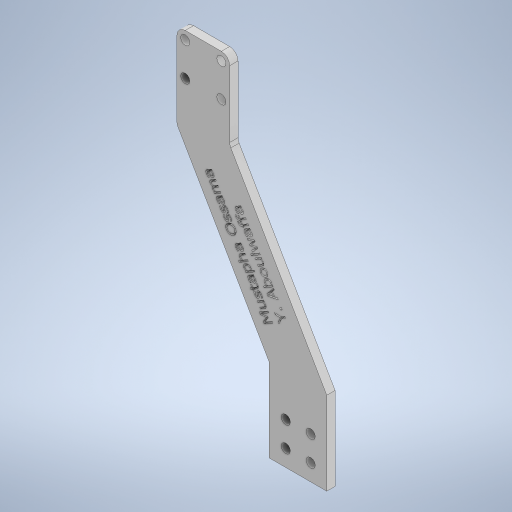
# Autodesk Inventor part: Arm
Saved by Autodesk Inventor 2023 (Build 270158000, 158)
## iProperties
Created: 2023-12-17
Part Number: Arm
Material: Generic
Document SubType Name: Modeling
Designer: Mustapha
Density: 1 g/cm^3
Appearance: Default
Author: Mustapha
Autodesk Inventor part; units mm, degrees
ref_plane "YZ Plane" through (0, 0, 0) normal (1, 0, 0) x (0, 1, 0)
ref_plane "XZ Plane" through (0, 0, 0) normal (0, 1, 0) x (-1, 0, 0)
ref_plane "XY Plane" through (0, 0, 0) normal (0, 0, 1) x (1, 0, 0)
sketch "Sketch1" plane through (0, 0, 0) normal (0, 0, 1) x (1, 0, 0)
  line L0 (0, 0) -> (-54.8483, 95)
  line L1 (-55.5181, 97.5) -> (-55.5181, 142.5)
  line L2 (-50.5181, 147.5) -> (-28.7639, 147.5)
  line L3 (-23.7639, 142.5) -> (-23.7639, 102.5)
  line L4 (-23.094, 100) -> (34.641, 0)
  line L5 (34.641, 0) -> (0, 0)
  arc A0 (-55.5181, 97.5) -> (-54.8483, 95) centre (-50.5181, 97.5) ccw
  arc A1 (-23.7639, 102.5) -> (-23.094, 100) centre (-18.7639, 102.5) ccw
  arc A2 (-23.7639, 142.5) -> (-28.7639, 147.5) centre (-28.7639, 142.5) ccw
  arc A3 (-50.5181, 147.5) -> (-55.5181, 142.5) centre (-50.5181, 142.5) ccw
  line L6 (0, 0) -> (0, -50)
  line L7 (0, -50) -> (34.641, -50)
  line L8 (34.641, -50) -> (34.641, 0)
  circle A4 centre (10, -40) radius 2.75
  circle A5 centre (25, -40) radius 2.75
  circle A6 centre (25, -25) radius 2.75
  circle A7 centre (10, -25) radius 2.75
  circle A8 centre (-50.5181, 142.5) radius 2.75
  circle A9 centre (-28.7639, 142.5) radius 2.75
  circle A10 centre (-50.5181, 122.5) radius 2.75
  circle A11 centre (-28.7639, 122.5) radius 2.75
  point P0 (-55.5181, 147.5)
  dimension "d0" = 5
  dimension "d1" = 30
  dimension "d2" = 50
  dimension "d3" = 5
  dimension "d4" = 50
  dimension "d5" = 40
  dimension "d6" = 100
  dimension "d7" = 120
  dimension "d8" = 5.5
  dimension "d11" = 15
  dimension "d18" = 15
  dimension "d23" = 10
  dimension "d24" = 10
  dimension "d25" = 5.5
  dimension "d26" = 5.5
  dimension "d29" = 20
  constraints: 18 end point, 12 centre point, 8 point on circle, 8 tangent, 5 perpendicular, 4 vertical, 2 coincident, 2 equal radius, 2 point on line, 1 horizontal, 1 parallel, 10 other
  measures "d0" radius of A0
  measures "d1" distance between parallel lines of L0 L4
  measures "d2" distance of L1.start point (-55.518, 147.5)
  measures "d3" radius of A2
  measures "d4" distance of L7.end L4.end
  measures "d5" distance of L3.start L3.end
  measures "d6" vertical distance of L4.start L4.end
  measures "d7" angle of L5 L0
  measures "d8" diameter of A4
  measures "d11" distance of A4.centre A5.centre
  measures "d18" distance of A5.centre A6.centre
  measures "d23" distance from line of L6 A7.centre
  measures "d24" distance from line of L7 A4.centre
  measures "d25" diameter of A8
  measures "d26" diameter of A9
  measures "d29" distance of A8.centre A10.centre
extrude "Extrusion1" add sketch "Sketch1" along normal blind 5
sketch "Sketch2" plane through (0, 0, 5) normal (0, 0, 1) x (1, 0, 0)
  line L0 (-2.8825, 17.5693) -> (-72.8343, 134.7749) construction
  line L1 (-72.8343, 134.7749) -> (-26.5058, 162.4251) construction
  line L2 (-26.5058, 162.4251) -> (43.446, 45.2195) construction
  line L3 (43.446, 45.2195) -> (-2.8825, 17.5693) construction
  line L4 (-0.7401, 26.209) -> (-0.2916, 25.4575)
  line L5 (-0.2916, 25.4575) -> (-4.7298, 22.8086)
  line L6 (-4.7298, 22.8086) -> (-0.8315, 23.1364)
  line L7 (-0.8315, 23.1364) -> (-0.5599, 22.6813)
  line L8 (-0.5599, 22.6813) -> (-2.7039, 19.4142)
  line L9 (-2.7039, 19.4142) -> (1.7343, 22.0631)
  line L10 (1.7343, 22.0631) -> (2.1554, 21.3575)
  line L11 (2.1554, 21.3575) -> (-2.9967, 18.2825)
  line L12 (-2.9967, 18.2825) -> (-3.6097, 19.3096)
  line L13 (-3.6097, 19.3096) -> (-1.5861, 22.4369)
  line L14 (-1.5861, 22.4369) -> (-5.2693, 22.0903)
  line L15 (-5.2693, 22.0903) -> (-5.8923, 23.1341)
  line L16 (-5.8923, 23.1341) -> (-0.7401, 26.209)
  line L17 (-3.369, 30.6138) -> (-2.9429, 29.8999)
  line L18 (-2.9429, 29.8999) -> (-3.3688, 29.6457)
  spline S0 degree 2 poles (-3.3688, 29.6457) (-2.9089, 29.4728) (-2.2812, 29.0378) (-2.0644, 28.6745) knots 0 0 0 1 2 2 2
  spline S1 degree 2 poles (-2.0644, 28.6745) (-1.8974, 28.3948) (-1.7729, 27.8066) (-1.8428, 27.5158) knots 0 0 0 1 2 2 2
  spline S2 degree 2 poles (-1.8428, 27.5158) (-1.9127, 27.2249) (-2.34, 26.6981) (-2.7325, 26.4638) knots 0 0 0 1 2 2 2
  line L19 (-2.7325, 26.4638) -> (-5.2418, 24.9662)
  line L20 (-5.2418, 24.9662) -> (-5.6679, 25.6802)
  line L21 (-5.6679, 25.6802) -> (-3.4634, 26.9959)
  spline S3 degree 2 poles (-3.4634, 26.9959) (-3.1544, 27.1803) (-2.7793, 27.4721) (-2.6814, 27.6495) knots 0 0 0 1 2 2 2
  spline S4 degree 2 poles (-2.6814, 27.6495) (-2.5834, 27.8269) (-2.625, 28.2097) (-2.792, 28.4894) knots 0 0 0 1 2 2 2
  spline S5 degree 2 poles (-2.792, 28.4894) (-2.949, 28.7525) (-3.5767, 29.1875) (-3.9199, 29.3168) knots 0 0 0 1 2 2 2
  line L22 (-3.9199, 29.3168) -> (-6.8091, 27.5924)
  line L23 (-6.8091, 27.5924) -> (-7.2352, 28.3063)
  line L24 (-7.2352, 28.3063) -> (-3.369, 30.6138)
  spline S6 degree 2 poles (-4.5804, 32.8522) (-4.3263, 32.4264) (-4.0915, 31.5586) (-4.0639, 31.2467) knots 0 0 0 1 2 2 2
  line L25 (-4.0639, 31.2467) -> (-4.7945, 30.8106)
  line L26 (-4.7945, 30.8106) -> (-4.8169, 30.8482)
  spline S7 degree 2 poles (-4.8169, 30.8482) (-4.805, 30.9799) (-4.7933, 31.3209) (-4.8277, 31.5778) knots 0 0 0 1 2 2 2
  spline S8 degree 2 poles (-4.8277, 31.5778) (-4.8581, 31.8089) (-5.0028, 32.3171) (-5.1423, 32.5509) knots 0 0 0 1 2 2 2
  spline S9 degree 2 poles (-5.1423, 32.5509) (-5.2445, 32.722) (-5.5514, 33.0655) (-5.663, 33.1291) knots 0 0 0 1 2 2 2
  spline S10 degree 2 poles (-5.663, 33.1291) (-5.8221, 33.2154) (-6.0714, 33.2251) (-6.2551, 33.1155) knots 0 0 0 1 2 2 2
  spline S11 degree 2 poles (-6.2551, 33.1155) (-6.4889, 32.9759) (-6.5582, 32.5608) (-6.4257, 32.1586) knots 0 0 0 1 2 2 2
  spline S12 degree 2 poles (-6.4257, 32.1586) (-6.3769, 32.0009) (-6.1946, 31.5151) (-6.1284, 31.2999) knots 0 0 0 1 2 2 2
  spline S13 degree 2 poles (-6.1284, 31.2999) (-5.9688, 30.7383) (-6.239, 29.9768) (-6.6232, 29.7475) knots 0 0 0 1 2 2 2
  spline S14 degree 2 poles (-6.6232, 29.7475) (-7.1451, 29.436) (-8.3189, 29.9132) (-8.7475, 30.6314) knots 0 0 0 1 2 2 2
  spline S15 degree 2 poles (-8.7475, 30.6314) (-8.9568, 30.9821) (-9.2267, 31.7949) (-9.2502, 32.1093) knots 0 0 0 1 2 2 2
  line L27 (-9.2502, 32.1093) -> (-8.5529, 32.5255)
  line L28 (-8.5529, 32.5255) -> (-8.5305, 32.4879)
  spline S16 degree 2 poles (-8.5305, 32.4879) (-8.5664, 32.0927) (-8.3949, 31.2835) (-8.1905, 30.9411) knots 0 0 0 1 2 2 2
  spline S17 degree 2 poles (-8.1905, 30.9411) (-7.9812, 30.5904) (-7.4183, 30.2639) (-7.1469, 30.4258) knots 0 0 0 1 2 2 2
  spline S18 degree 2 poles (-7.1469, 30.4258) (-6.9006, 30.5729) (-6.8345, 31.003) (-6.9488, 31.3651) knots 0 0 0 1 2 2 2
  spline S19 degree 2 poles (-6.9488, 31.3651) (-7.0084, 31.5504) (-7.165, 31.9835) (-7.2486, 32.2281) knots 0 0 0 1 2 2 2
  spline S20 degree 2 poles (-7.2486, 32.2281) (-7.4216, 32.7646) (-7.2089, 33.5371) (-6.7788, 33.7938) knots 0 0 0 1 2 2 2
  spline S21 degree 2 poles (-6.7788, 33.7938) (-6.5283, 33.9433) (-5.9562, 33.9904) (-5.6687, 33.8788) knots 0 0 0 1 2 2 2
  spline S22 degree 2 poles (-5.6687, 33.8788) (-5.3605, 33.7513) (-4.8396, 33.2865) (-4.5804, 32.8522) knots 0 0 0 1 2 2 2
  spline S23 degree 2 poles (-6.7551, 36.458) (-6.4062, 35.8734) (-6.6204, 34.8566) (-7.2759, 34.4654) knots 0 0 0 1 2 2 2
  line L29 (-7.2759, 34.4654) -> (-9.4178, 33.1871)
  line L30 (-9.4178, 33.1871) -> (-9.1287, 32.7028)
  line L31 (-9.1287, 32.7028) -> (-9.6673, 32.3813)
  line L32 (-9.6673, 32.3813) -> (-9.9564, 32.8656)
  line L33 (-9.9564, 32.8656) -> (-11.067, 32.2028)
  line L34 (-11.067, 32.2028) -> (-11.4931, 32.9167)
  line L35 (-11.4931, 32.9167) -> (-10.3825, 33.5796)
  line L36 (-10.3825, 33.5796) -> (-11.1674, 34.8948)
  line L37 (-11.1674, 34.8948) -> (-10.6288, 35.2162)
  line L38 (-10.6288, 35.2162) -> (-9.8439, 33.901)
  line L39 (-9.8439, 33.901) -> (-8.0026, 34.9999)
  spline S24 degree 2 poles (-8.0026, 34.9999) (-7.7104, 35.1744) (-7.4013, 35.3871) (-7.3109, 35.5487) knots 0 0 0 1 2 2 2
  spline S25 degree 2 poles (-7.3109, 35.5487) (-7.2272, 35.6836) (-7.2781, 36.0439) (-7.4276, 36.2944) knots 0 0 0 1 2 2 2
  spline S26 degree 2 poles (-7.4276, 36.2944) (-7.5297, 36.4656) (-7.8226, 36.7381) (-7.8942, 36.7917) knots 0 0 0 1 2 2 2
  line L40 (-7.8942, 36.7917) -> (-7.9191, 36.8334)
  line L41 (-7.9191, 36.8334) -> (-7.3346, 37.1823)
  spline S27 degree 2 poles (-7.3346, 37.1823) (-7.1649, 37.0118) (-6.8597, 36.6333) (-6.7551, 36.458) knots 0 0 0 1 2 2 2
  spline S28 degree 2 poles (-9.4397, 39.8556) (-9.3289, 39.8028) (-8.9458, 39.6351) (-8.8009, 39.5347) knots 0 0 0 1 2 2 2
  spline S29 degree 2 poles (-8.8009, 39.5347) (-8.5969, 39.4017) (-8.2891, 39.1041) (-8.0997, 38.7868) knots 0 0 0 1 2 2 2
  spline S30 degree 2 poles (-8.0997, 38.7868) (-7.9427, 38.5237) (-7.8407, 37.9448) (-7.8963, 37.6681) knots 0 0 0 1 2 2 2
  spline S31 degree 2 poles (-7.8963, 37.6681) (-7.9528, 37.4022) (-8.2983, 36.9185) (-8.5572, 36.764) knots 0 0 0 1 2 2 2
  spline S32 degree 2 poles (-8.5572, 36.764) (-8.958, 36.5248) (-9.7476, 36.5575) (-10.1522, 36.8653) knots 0 0 0 1 2 2 2
  spline S33 degree 2 poles (-10.1522, 36.8653) (-10.5143, 37.1305) (-11.2076, 38.036) (-11.5732, 38.5822) knots 0 0 0 1 2 2 2
  line L42 (-11.5732, 38.5822) -> (-11.6985, 38.5075)
  spline S34 degree 2 poles (-11.6985, 38.5075) (-11.9239, 38.3729) (-12.114, 38.0557) (-12.1111, 37.8705) knots 0 0 0 1 2 2 2
  spline S35 degree 2 poles (-12.1111, 37.8705) (-12.1082, 37.6854) (-11.9215, 37.2589) (-11.7969, 37.0501) knots 0 0 0 1 2 2 2
  spline S36 degree 2 poles (-11.7969, 37.0501) (-11.6499, 36.8038) (-11.1176, 36.2155) (-10.7888, 35.9587) knots 0 0 0 1 2 2 2
  line L43 (-10.7888, 35.9587) -> (-10.7639, 35.917)
  line L44 (-10.7639, 35.917) -> (-11.4278, 35.5208)
  spline S37 degree 2 poles (-11.4278, 35.5208) (-11.595, 35.6871) (-12.1613, 36.3513) (-12.3781, 36.7146) knots 0 0 0 1 2 2 2
  spline S38 degree 2 poles (-12.3781, 36.7146) (-12.6373, 37.1488) (-12.8708, 37.8248) (-12.8525, 38.1641) knots 0 0 0 1 2 2 2
  spline S39 degree 2 poles (-12.8525, 38.1641) (-12.8309, 38.4884) (-12.4628, 39.0196) (-12.0995, 39.2364) knots 0 0 0 1 2 2 2
  line L45 (-12.0995, 39.2364) -> (-9.4567, 40.8137)
  line L46 (-9.4567, 40.8137) -> (-9.0306, 40.0998)
  line L47 (-9.0306, 40.0998) -> (-9.4397, 39.8556)
  line L48 (-9.9825, 39.5316) -> (-11.0555, 38.8912)
  spline S40 degree 2 poles (-11.0555, 38.8912) (-10.8826, 38.649) (-10.3482, 37.9148) (-10.1368, 37.7125) knots 0 0 0 1 2 2 2
  spline S41 degree 2 poles (-10.1368, 37.7125) (-9.8881, 37.4759) (-9.3364, 37.3012) (-9.0442, 37.4756) knots 0 0 0 1 2 2 2
  spline S42 degree 2 poles (-9.0442, 37.4756) (-8.7102, 37.675) (-8.6162, 38.286) (-8.8529, 38.6826) knots 0 0 0 1 2 2 2
  spline S43 degree 2 poles (-8.8529, 38.6826) (-9.0548, 39.0208) (-9.6442, 39.4108) (-9.9825, 39.5316) knots 0 0 0 1 2 2 2
  spline S44 degree 2 poles (-14.2202, 44.1653) (-13.2516, 44.7434) (-11.5021, 44.4117) (-11.0386, 43.6351) knots 0 0 0 1 2 2 2
  spline S45 degree 2 poles (-11.0386, 43.6351) (-10.8517, 43.3219) (-10.6938, 42.7537) (-10.6795, 42.4168) knots 0 0 0 1 2 2 2
  line L49 (-10.6795, 42.4168) -> (-9.0596, 43.3836)
  line L50 (-9.0596, 43.3836) -> (-8.6335, 42.6697)
  line L51 (-8.6335, 42.6697) -> (-13.9234, 39.5125)
  line L52 (-13.9234, 39.5125) -> (-14.3495, 40.2264)
  line L53 (-14.3495, 40.2264) -> (-13.9445, 40.4681)
  spline S46 degree 2 poles (-13.9445, 40.4681) (-14.3253, 40.6033) (-15.0038, 41.076) (-15.233, 41.4601) knots 0 0 0 1 2 2 2
  spline S47 degree 2 poles (-15.233, 41.4601) (-15.6691, 42.1908) (-15.1054, 43.6371) (-14.2202, 44.1653) knots 0 0 0 1 2 2 2
  spline S48 degree 2 poles (-13.704, 43.4712) (-14.3679, 43.075) (-14.8219, 42.1755) (-14.5105, 41.6536) knots 0 0 0 1 2 2 2
  spline S49 degree 2 poles (-14.5105, 41.6536) (-14.331, 41.353) (-13.7458, 40.9321) (-13.4017, 40.7921) knots 0 0 0 1 2 2 2
  line L54 (-13.4017, 40.7921) -> (-11.2056, 42.1028)
  spline S50 degree 2 poles (-11.2056, 42.1028) (-11.2515, 42.4548) (-11.3989, 42.9104) (-11.5533, 43.1693) knots 0 0 0 1 2 2 2
  spline S51 degree 2 poles (-11.5533, 43.1693) (-11.8848, 43.7246) (-12.9942, 43.8948) (-13.704, 43.4712) knots 0 0 0 1 2 2 2
  line L55 (-14.6198, 49.4647) -> (-14.1937, 48.7507)
  line L56 (-14.1937, 48.7507) -> (-16.3982, 47.435)
  spline S52 degree 2 poles (-16.3982, 47.435) (-16.6654, 47.2755) (-17.0898, 46.943) (-17.1802, 46.7814) knots 0 0 0 1 2 2 2
  spline S53 degree 2 poles (-17.1802, 46.7814) (-17.274, 46.6065) (-17.2291, 46.2087) (-17.0696, 45.9415) knots 0 0 0 1 2 2 2
  spline S54 degree 2 poles (-17.0696, 45.9415) (-16.9101, 45.6742) (-16.3124, 45.2609) (-15.9416, 45.1141) knots 0 0 0 1 2 2 2
  line L57 (-15.9416, 45.1141) -> (-13.0524, 46.8385)
  line L58 (-13.0524, 46.8385) -> (-12.6263, 46.1245)
  line L59 (-12.6263, 46.1245) -> (-18.0081, 42.9125)
  line L60 (-18.0081, 42.9125) -> (-18.4342, 43.6265)
  line L61 (-18.4342, 43.6265) -> (-16.4886, 44.7877)
  spline S55 degree 2 poles (-16.4886, 44.7877) (-16.9435, 44.9522) (-17.5903, 45.4098) (-17.7972, 45.7564) knots 0 0 0 1 2 2 2
  spline S56 degree 2 poles (-17.7972, 45.7564) (-18.1709, 46.3826) (-17.843, 47.541) (-17.1291, 47.9671) knots 0 0 0 1 2 2 2
  line L62 (-17.1291, 47.9671) -> (-14.6198, 49.4647)
  spline S57 degree 2 poles (-17.0424, 52.594) (-16.9316, 52.5412) (-16.5484, 52.3735) (-16.4036, 52.2731) knots 0 0 0 1 2 2 2
  spline S58 degree 2 poles (-16.4036, 52.2731) (-16.1996, 52.1401) (-15.8917, 51.8425) (-15.7024, 51.5252) knots 0 0 0 1 2 2 2
  spline S59 degree 2 poles (-15.7024, 51.5252) (-15.5454, 51.2622) (-15.4433, 50.6832) (-15.499, 50.4065) knots 0 0 0 1 2 2 2
  spline S60 degree 2 poles (-15.499, 50.4065) (-15.5555, 50.1406) (-15.901, 49.6569) (-16.1599, 49.5025) knots 0 0 0 1 2 2 2
  spline S61 degree 2 poles (-16.1599, 49.5025) (-16.5607, 49.2632) (-17.3503, 49.2959) (-17.7548, 49.6037) knots 0 0 0 1 2 2 2
  spline S62 degree 2 poles (-17.7548, 49.6037) (-18.1169, 49.8689) (-18.8103, 50.7745) (-19.1759, 51.3207) knots 0 0 0 1 2 2 2
  line L63 (-19.1759, 51.3207) -> (-19.3011, 51.2459)
  spline S63 degree 2 poles (-19.3011, 51.2459) (-19.5266, 51.1113) (-19.7166, 50.7941) (-19.7137, 50.609) knots 0 0 0 1 2 2 2
  spline S64 degree 2 poles (-19.7137, 50.609) (-19.7108, 50.4238) (-19.5242, 49.9973) (-19.3996, 49.7885) knots 0 0 0 1 2 2 2
  spline S65 degree 2 poles (-19.3996, 49.7885) (-19.2526, 49.5422) (-18.7203, 48.9539) (-18.3915, 48.6971) knots 0 0 0 1 2 2 2
  line L64 (-18.3915, 48.6971) -> (-18.3666, 48.6554)
  line L65 (-18.3666, 48.6554) -> (-19.0304, 48.2592)
  spline S66 degree 2 poles (-19.0304, 48.2592) (-19.1977, 48.4255) (-19.764, 49.0898) (-19.9808, 49.453) knots 0 0 0 1 2 2 2
  spline S67 degree 2 poles (-19.9808, 49.453) (-20.2399, 49.8872) (-20.4735, 50.5632) (-20.4552, 50.9025) knots 0 0 0 1 2 2 2
  spline S68 degree 2 poles (-20.4552, 50.9025) (-20.4336, 51.2269) (-20.0654, 51.758) (-19.7022, 51.9748) knots 0 0 0 1 2 2 2
  line L66 (-19.7022, 51.9748) -> (-17.0593, 53.5522)
  line L67 (-17.0593, 53.5522) -> (-16.6332, 52.8382)
  line L68 (-16.6332, 52.8382) -> (-17.0424, 52.594)
  line L69 (-17.5852, 52.2701) -> (-18.6582, 51.6296)
  spline S69 degree 2 poles (-18.6582, 51.6296) (-18.4853, 51.3874) (-17.9508, 50.6532) (-17.7395, 50.4509) knots 0 0 0 1 2 2 2
  spline S70 degree 2 poles (-17.7395, 50.4509) (-17.4907, 50.2143) (-16.9391, 50.0396) (-16.6469, 50.214) knots 0 0 0 1 2 2 2
  spline S71 degree 2 poles (-16.6469, 50.214) (-16.3128, 50.4134) (-16.2189, 51.0244) (-16.4556, 51.421) knots 0 0 0 1 2 2 2
  spline S72 degree 2 poles (-16.4556, 51.421) (-16.6574, 51.7592) (-17.2469, 52.1492) (-17.5852, 52.2701) knots 0 0 0 1 2 2 2
  spline S73 degree 2 poles (-26.1007, 58.3313) (-25.9502, 58.8571) (-25.1624, 59.8142) (-24.5194, 60.198) knots 0 0 0 1 2 2 2
  spline S74 degree 2 poles (-24.5194, 60.198) (-23.8932, 60.5718) (-22.6693, 60.8266) (-22.1301, 60.7011) knots 0 0 0 1 2 2 2
  spline S75 degree 2 poles (-22.1301, 60.7011) (-21.5642, 60.5688) (-20.6711, 59.8505) (-20.3397, 59.2952) knots 0 0 0 1 2 2 2
  spline S76 degree 2 poles (-20.3397, 59.2952) (-19.9958, 58.719) (-19.8, 57.5845) (-19.9497, 57.0478) knots 0 0 0 1 2 2 2
  spline S77 degree 2 poles (-19.9497, 57.0478) (-20.0977, 56.5178) (-20.8946, 55.5666) (-21.5292, 55.1878) knots 0 0 0 1 2 2 2
  spline S78 degree 2 poles (-21.5292, 55.1878) (-22.1764, 54.8016) (-23.3735, 54.5684) (-23.9228, 54.6822) knots 0 0 0 1 2 2 2
  spline S79 degree 2 poles (-23.9228, 54.6822) (-24.4595, 54.8036) (-25.3676, 55.5186) (-25.709, 56.0906) knots 0 0 0 1 2 2 2
  spline S80 degree 2 poles (-25.709, 56.0906) (-26.0528, 56.6668) (-26.2386, 57.813) (-26.1007, 58.3313) knots 0 0 0 1 2 2 2
  spline S81 degree 2 poles (-24.051, 59.4131) (-24.5603, 59.1091) (-25.2049, 58.3959) (-25.3317, 58.0202) knots 0 0 0 1 2 2 2
  spline S82 degree 2 poles (-25.3317, 58.0202) (-25.4644, 57.6352) (-25.3528, 56.8411) (-25.1161, 56.4445) knots 0 0 0 1 2 2 2
  spline S83 degree 2 poles (-25.1161, 56.4445) (-24.8719, 56.0353) (-24.2492, 55.5802) (-23.8316, 55.5067) knots 0 0 0 1 2 2 2
  spline S84 degree 2 poles (-23.8316, 55.5067) (-23.434, 55.4382) (-22.4987, 55.6737) (-21.9977, 55.9727) knots 0 0 0 1 2 2 2
  spline S85 degree 2 poles (-21.9977, 55.9727) (-20.9831, 56.5783) (-20.4641, 58.1564) (-20.9326, 58.9413) knots 0 0 0 1 2 2 2
  spline S86 degree 2 poles (-20.9326, 58.9413) (-21.4035, 59.7304) (-23.0364, 60.0186) (-24.051, 59.4131) knots 0 0 0 1 2 2 2
  spline S87 degree 2 poles (-22.9953, 63.7067) (-22.7411, 63.2808) (-22.5063, 62.4131) (-22.4787, 62.1011) knots 0 0 0 1 2 2 2
  line L70 (-22.4787, 62.1011) -> (-23.2094, 61.665)
  line L71 (-23.2094, 61.665) -> (-23.2318, 61.7026)
  spline S88 degree 2 poles (-23.2318, 61.7026) (-23.2198, 61.8343) (-23.2082, 62.1754) (-23.2426, 62.4323) knots 0 0 0 1 2 2 2
  spline S89 degree 2 poles (-23.2426, 62.4323) (-23.2729, 62.6633) (-23.4176, 63.1715) (-23.5572, 63.4053) knots 0 0 0 1 2 2 2
  spline S90 degree 2 poles (-23.5572, 63.4053) (-23.6593, 63.5765) (-23.9662, 63.9199) (-24.0778, 63.9836) knots 0 0 0 1 2 2 2
  spline S91 degree 2 poles (-24.0778, 63.9836) (-24.2369, 64.0698) (-24.4862, 64.0796) (-24.6699, 63.9699) knots 0 0 0 1 2 2 2
  spline S92 degree 2 poles (-24.6699, 63.9699) (-24.9037, 63.8304) (-24.9731, 63.4153) (-24.8406, 63.0131) knots 0 0 0 1 2 2 2
  spline S93 degree 2 poles (-24.8406, 63.0131) (-24.7918, 62.8553) (-24.6094, 62.3696) (-24.5432, 62.1543) knots 0 0 0 1 2 2 2
  spline S94 degree 2 poles (-24.5432, 62.1543) (-24.3836, 61.5927) (-24.6539, 60.8312) (-25.038, 60.602) knots 0 0 0 1 2 2 2
  spline S95 degree 2 poles (-25.038, 60.602) (-25.5599, 60.2905) (-26.7337, 60.7677) (-27.1623, 61.4858) knots 0 0 0 1 2 2 2
  spline S96 degree 2 poles (-27.1623, 61.4858) (-27.3716, 61.8365) (-27.6416, 62.6494) (-27.665, 62.9638) knots 0 0 0 1 2 2 2
  line L72 (-27.665, 62.9638) -> (-26.9678, 63.3799)
  line L73 (-26.9678, 63.3799) -> (-26.9453, 63.3423)
  spline S97 degree 2 poles (-26.9453, 63.3423) (-26.9813, 62.9472) (-26.8097, 62.1379) (-26.6054, 61.7956) knots 0 0 0 1 2 2 2
  spline S98 degree 2 poles (-26.6054, 61.7956) (-26.3961, 61.4448) (-25.8331, 61.1183) (-25.5618, 61.2803) knots 0 0 0 1 2 2 2
  spline S99 degree 2 poles (-25.5618, 61.2803) (-25.3154, 61.4273) (-25.2494, 61.8574) (-25.3636, 62.2196) knots 0 0 0 1 2 2 2
  spline S100 degree 2 poles (-25.3636, 62.2196) (-25.4232, 62.4049) (-25.5798, 62.838) (-25.6635, 63.0825) knots 0 0 0 1 2 2 2
  spline S101 degree 2 poles (-25.6635, 63.0825) (-25.8365, 63.6191) (-25.6237, 64.3916) (-25.1937, 64.6483) knots 0 0 0 1 2 2 2
  spline S102 degree 2 poles (-25.1937, 64.6483) (-24.9432, 64.7978) (-24.371, 64.8448) (-24.0836, 64.7332) knots 0 0 0 1 2 2 2
  spline S103 degree 2 poles (-24.0836, 64.7332) (-23.7754, 64.6058) (-23.2544, 64.1409) (-22.9953, 63.7067) knots 0 0 0 1 2 2 2
  spline S104 degree 2 poles (-25.071, 67.1846) (-24.8168, 66.7587) (-24.582, 65.891) (-24.5544, 65.579) knots 0 0 0 1 2 2 2
  line L74 (-24.5544, 65.579) -> (-25.2851, 65.143)
  line L75 (-25.2851, 65.143) -> (-25.3075, 65.1805)
  spline S105 degree 2 poles (-25.3075, 65.1805) (-25.2955, 65.3123) (-25.2839, 65.6533) (-25.3183, 65.9102) knots 0 0 0 1 2 2 2
  spline S106 degree 2 poles (-25.3183, 65.9102) (-25.3486, 66.1412) (-25.4934, 66.6494) (-25.6329, 66.8832) knots 0 0 0 1 2 2 2
  spline S107 degree 2 poles (-25.6329, 66.8832) (-25.7351, 67.0544) (-26.042, 67.3978) (-26.1536, 67.4615) knots 0 0 0 1 2 2 2
  spline S108 degree 2 poles (-26.1536, 67.4615) (-26.3126, 67.5477) (-26.5619, 67.5575) (-26.7456, 67.4478) knots 0 0 0 1 2 2 2
  spline S109 degree 2 poles (-26.7456, 67.4478) (-26.9794, 67.3083) (-27.0488, 66.8932) (-26.9163, 66.491) knots 0 0 0 1 2 2 2
  spline S110 degree 2 poles (-26.9163, 66.491) (-26.8675, 66.3332) (-26.6852, 65.8475) (-26.619, 65.6322) knots 0 0 0 1 2 2 2
  spline S111 degree 2 poles (-26.619, 65.6322) (-26.4593, 65.0707) (-26.7296, 64.3091) (-27.1137, 64.0799) knots 0 0 0 1 2 2 2
  spline S112 degree 2 poles (-27.1137, 64.0799) (-27.6356, 63.7684) (-28.8094, 64.2456) (-29.238, 64.9637) knots 0 0 0 1 2 2 2
  spline S113 degree 2 poles (-29.238, 64.9637) (-29.4473, 65.3144) (-29.7173, 66.1273) (-29.7407, 66.4417) knots 0 0 0 1 2 2 2
  line L76 (-29.7407, 66.4417) -> (-29.0435, 66.8578)
  line L77 (-29.0435, 66.8578) -> (-29.0211, 66.8203)
  spline S114 degree 2 poles (-29.0211, 66.8203) (-29.057, 66.4251) (-28.8854, 65.6158) (-28.6811, 65.2735) knots 0 0 0 1 2 2 2
  spline S115 degree 2 poles (-28.6811, 65.2735) (-28.4718, 64.9228) (-27.9089, 64.5962) (-27.6375, 64.7582) knots 0 0 0 1 2 2 2
  spline S116 degree 2 poles (-27.6375, 64.7582) (-27.3911, 64.9052) (-27.3251, 65.3353) (-27.4393, 65.6975) knots 0 0 0 1 2 2 2
  spline S117 degree 2 poles (-27.4393, 65.6975) (-27.4989, 65.8828) (-27.6555, 66.3159) (-27.7392, 66.5604) knots 0 0 0 1 2 2 2
  spline S118 degree 2 poles (-27.7392, 66.5604) (-27.9122, 67.097) (-27.6994, 67.8695) (-27.2694, 68.1262) knots 0 0 0 1 2 2 2
  spline S119 degree 2 poles (-27.2694, 68.1262) (-27.0189, 68.2757) (-26.4467, 68.3227) (-26.1593, 68.2111) knots 0 0 0 1 2 2 2
  spline S120 degree 2 poles (-26.1593, 68.2111) (-25.8511, 68.0837) (-25.3302, 67.6188) (-25.071, 67.1846) knots 0 0 0 1 2 2 2
  spline S121 degree 2 poles (-28.3754, 71.5826) (-28.2646, 71.5298) (-27.8814, 71.3622) (-27.7365, 71.2618) knots 0 0 0 1 2 2 2
  spline S122 degree 2 poles (-27.7365, 71.2618) (-27.5326, 71.1287) (-27.2247, 70.8311) (-27.0353, 70.5138) knots 0 0 0 1 2 2 2
  spline S123 degree 2 poles (-27.0353, 70.5138) (-26.8783, 70.2508) (-26.7763, 69.6718) (-26.832, 69.3951) knots 0 0 0 1 2 2 2
  spline S124 degree 2 poles (-26.832, 69.3951) (-26.8885, 69.1293) (-27.234, 68.6456) (-27.4928, 68.4911) knots 0 0 0 1 2 2 2
  spline S125 degree 2 poles (-27.4928, 68.4911) (-27.8937, 68.2519) (-28.6833, 68.2846) (-29.0878, 68.5924) knots 0 0 0 1 2 2 2
  spline S126 degree 2 poles (-29.0878, 68.5924) (-29.4499, 68.8576) (-30.1432, 69.7631) (-30.5089, 70.3093) knots 0 0 0 1 2 2 2
  line L78 (-30.5089, 70.3093) -> (-30.6341, 70.2345)
  spline S127 degree 2 poles (-30.6341, 70.2345) (-30.8596, 70.1) (-31.0496, 69.7827) (-31.0467, 69.5976) knots 0 0 0 1 2 2 2
  spline S128 degree 2 poles (-31.0467, 69.5976) (-31.0438, 69.4125) (-30.8572, 68.9859) (-30.7326, 68.7772) knots 0 0 0 1 2 2 2
  spline S129 degree 2 poles (-30.7326, 68.7772) (-30.5856, 68.5308) (-30.0533, 67.9425) (-29.7245, 67.6858) knots 0 0 0 1 2 2 2
  line L79 (-29.7245, 67.6858) -> (-29.6996, 67.644)
  line L80 (-29.6996, 67.644) -> (-30.3634, 67.2478)
  spline S130 degree 2 poles (-30.3634, 67.2478) (-30.5306, 67.4142) (-31.097, 68.0784) (-31.3137, 68.4416) knots 0 0 0 1 2 2 2
  spline S131 degree 2 poles (-31.3137, 68.4416) (-31.5729, 68.8759) (-31.8065, 69.5518) (-31.7882, 69.8912) knots 0 0 0 1 2 2 2
  spline S132 degree 2 poles (-31.7882, 69.8912) (-31.7666, 70.2155) (-31.3984, 70.7467) (-31.0352, 70.9634) knots 0 0 0 1 2 2 2
  line L81 (-31.0352, 70.9634) -> (-28.3923, 72.5408)
  line L82 (-28.3923, 72.5408) -> (-27.9662, 71.8268)
  line L83 (-27.9662, 71.8268) -> (-28.3754, 71.5826)
  line L84 (-28.9181, 71.2587) -> (-29.9912, 70.6183)
  spline S133 degree 2 poles (-29.9912, 70.6183) (-29.8183, 70.3761) (-29.2838, 69.6418) (-29.0725, 69.4396) knots 0 0 0 1 2 2 2
  spline S134 degree 2 poles (-29.0725, 69.4396) (-28.8237, 69.203) (-28.2721, 69.0283) (-27.9798, 69.2027) knots 0 0 0 1 2 2 2
  spline S135 degree 2 poles (-27.9798, 69.2027) (-27.6458, 69.402) (-27.5518, 70.013) (-27.7886, 70.4097) knots 0 0 0 1 2 2 2
  spline S136 degree 2 poles (-27.7886, 70.4097) (-27.9904, 70.7479) (-28.5799, 71.1378) (-28.9181, 71.2587) knots 0 0 0 1 2 2 2
  line L85 (-31.8734, 78.3735) -> (-34.1113, 77.0379)
  spline S137 degree 2 poles (-34.1113, 77.0379) (-34.3785, 76.8784) (-34.8062, 76.5608) (-34.8891, 76.4151) knots 0 0 0 1 2 2 2
  spline S138 degree 2 poles (-34.8891, 76.4151) (-34.9795, 76.2535) (-34.9462, 75.8941) (-34.8017, 75.6519) knots 0 0 0 1 2 2 2
  spline S139 degree 2 poles (-34.8017, 75.6519) (-34.6721, 75.4348) (-34.1217, 75.0725) (-33.726, 74.9406) knots 0 0 0 1 2 2 2
  spline S140 degree 2 poles (-33.726, 74.9406) (-33.67, 74.9797) (-33.5147, 75.0894) (-33.4061, 75.1542) knots 0 0 0 1 2 2 2
  line L86 (-33.4061, 75.1542) -> (-30.8592, 76.6742)
  line L87 (-30.8592, 76.6742) -> (-30.4331, 75.9602)
  line L88 (-30.4331, 75.9602) -> (-32.671, 74.6246)
  spline S141 degree 2 poles (-32.671, 74.6246) (-32.9382, 74.4651) (-33.3659, 74.1476) (-33.4488, 74.0019) knots 0 0 0 1 2 2 2
  spline S142 degree 2 poles (-33.4488, 74.0019) (-33.5392, 73.8403) (-33.5059, 73.4808) (-33.3614, 73.2387) knots 0 0 0 1 2 2 2
  spline S143 degree 2 poles (-33.3614, 73.2387) (-33.2243, 73.009) (-32.6548, 72.6525) (-32.3082, 72.5366) knots 0 0 0 1 2 2 2
  line L89 (-32.3082, 72.5366) -> (-29.419, 74.261)
  line L90 (-29.419, 74.261) -> (-28.9928, 73.547)
  line L91 (-28.9928, 73.547) -> (-32.859, 71.2395)
  line L92 (-32.859, 71.2395) -> (-33.2852, 71.9535)
  line L93 (-33.2852, 71.9535) -> (-32.8593, 72.2077)
  spline S144 degree 2 poles (-32.8593, 72.2077) (-33.2809, 72.3354) (-33.8921, 72.7237) (-34.0889, 73.0536) knots 0 0 0 1 2 2 2
  spline S145 degree 2 poles (-34.0889, 73.0536) (-34.3132, 73.4293) (-34.3489, 74.2008) (-34.0837, 74.5629) knots 0 0 0 1 2 2 2
  spline S146 degree 2 poles (-34.0837, 74.5629) (-34.6079, 74.6917) (-35.3124, 75.1036) (-35.5292, 75.4668) knots 0 0 0 1 2 2 2
  spline S147 degree 2 poles (-35.5292, 75.4668) (-35.6937, 75.7424) (-35.8058, 76.2813) (-35.7302, 76.553) knots 0 0 0 1 2 2 2
  spline S148 degree 2 poles (-35.7302, 76.553) (-35.657, 76.8288) (-35.243, 77.3307) (-34.8464, 77.5674) knots 0 0 0 1 2 2 2
  line L94 (-34.8464, 77.5674) -> (-32.2995, 79.0874)
  line L95 (-32.2995, 79.0874) -> (-31.8734, 78.3735)
  spline S149 degree 2 poles (-34.7196, 82.2126) (-34.6089, 82.1598) (-34.2257, 81.9921) (-34.0808, 81.8917) knots 0 0 0 1 2 2 2
  spline S150 degree 2 poles (-34.0808, 81.8917) (-33.8768, 81.7587) (-33.569, 81.4611) (-33.3796, 81.1438) knots 0 0 0 1 2 2 2
  spline S151 degree 2 poles (-33.3796, 81.1438) (-33.2226, 80.8808) (-33.1206, 80.3018) (-33.1763, 80.0251) knots 0 0 0 1 2 2 2
  spline S152 degree 2 poles (-33.1763, 80.0251) (-33.2327, 79.7592) (-33.5783, 79.2756) (-33.8371, 79.1211) knots 0 0 0 1 2 2 2
  spline S153 degree 2 poles (-33.8371, 79.1211) (-34.2379, 78.8818) (-35.0275, 78.9145) (-35.4321, 79.2223) knots 0 0 0 1 2 2 2
  spline S154 degree 2 poles (-35.4321, 79.2223) (-35.7942, 79.4875) (-36.4875, 80.3931) (-36.8532, 80.9393) knots 0 0 0 1 2 2 2
  line L96 (-36.8532, 80.9393) -> (-36.9784, 80.8645)
  spline S155 degree 2 poles (-36.9784, 80.8645) (-37.2039, 80.7299) (-37.3939, 80.4127) (-37.391, 80.2276) knots 0 0 0 1 2 2 2
  spline S156 degree 2 poles (-37.391, 80.2276) (-37.3881, 80.0424) (-37.2015, 79.6159) (-37.0769, 79.4071) knots 0 0 0 1 2 2 2
  spline S157 degree 2 poles (-37.0769, 79.4071) (-36.9298, 79.1608) (-36.3975, 78.5725) (-36.0688, 78.3157) knots 0 0 0 1 2 2 2
  line L97 (-36.0688, 78.3157) -> (-36.0438, 78.274)
  line L98 (-36.0438, 78.274) -> (-36.7077, 77.8778)
  spline S158 degree 2 poles (-36.7077, 77.8778) (-36.8749, 78.0441) (-37.4412, 78.7084) (-37.658, 79.0716) knots 0 0 0 1 2 2 2
  spline S159 degree 2 poles (-37.658, 79.0716) (-37.9172, 79.5058) (-38.1508, 80.1818) (-38.1324, 80.5211) knots 0 0 0 1 2 2 2
  spline S160 degree 2 poles (-38.1324, 80.5211) (-38.1108, 80.8455) (-37.7427, 81.3766) (-37.3795, 81.5934) knots 0 0 0 1 2 2 2
  line L99 (-37.3795, 81.5934) -> (-34.7366, 83.1708)
  line L100 (-34.7366, 83.1708) -> (-34.3105, 82.4568)
  line L101 (-34.3105, 82.4568) -> (-34.7196, 82.2126)
  line L102 (-35.2624, 81.8887) -> (-36.3354, 81.2483)
  spline S161 degree 2 poles (-36.3354, 81.2483) (-36.1626, 81.006) (-35.6281, 80.2718) (-35.4168, 80.0695) knots 0 0 0 1 2 2 2
  spline S162 degree 2 poles (-35.4168, 80.0695) (-35.168, 79.833) (-34.6164, 79.6582) (-34.3241, 79.8326) knots 0 0 0 1 2 2 2
  spline S163 degree 2 poles (-34.3241, 79.8326) (-33.9901, 80.032) (-33.8961, 80.643) (-34.1328, 81.0396) knots 0 0 0 1 2 2 2
  spline S164 degree 2 poles (-34.1328, 81.0396) (-34.3347, 81.3778) (-34.9241, 81.7678) (-35.2624, 81.8887) knots 0 0 0 1 2 2 2
  line L103 (3.1239, 27.3034) -> (7.1376, 27.1056)
  line L104 (7.1376, 27.1056) -> (9.4173, 28.4661)
  line L105 (9.4173, 28.4661) -> (9.8658, 27.7146)
  line L106 (9.8658, 27.7146) -> (7.6571, 26.3964)
  line L107 (7.6571, 26.3964) -> (5.8549, 22.7274)
  line L108 (5.8549, 22.7274) -> (5.3566, 23.5625)
  line L109 (5.3566, 23.5625) -> (6.7557, 26.3793)
  line L110 (6.7557, 26.3793) -> (3.5998, 26.506)
  line L111 (3.5998, 26.506) -> (3.1239, 27.3034)
  line L112 (7.3291, 31.9649) -> (7.8723, 31.0547)
  line L113 (7.8723, 31.0547) -> (6.887, 30.4667)
  line L114 (6.887, 30.4667) -> (6.3438, 31.3768)
  line L115 (6.3438, 31.3768) -> (7.3291, 31.9649)
  line L116 (5.4652, 35.0879) -> (-0.8257, 33.921)
  line L117 (-0.8257, 33.921) -> (-1.3814, 34.8521)
  line L118 (-1.3814, 34.8521) -> (2.6319, 39.8351)
  line L119 (2.6319, 39.8351) -> (3.1054, 39.0418)
  line L120 (3.1054, 39.0418) -> (1.9715, 37.6686)
  line L121 (1.9715, 37.6686) -> (3.2647, 35.5017)
  line L122 (3.2647, 35.5017) -> (5.0117, 35.8478)
  line L123 (5.0117, 35.8478) -> (5.4652, 35.0879)
  line L124 (1.5115, 37.111) -> (-0.3951, 34.7839)
  line L125 (-0.3951, 34.7839) -> (2.5531, 35.3658)
  line L126 (2.5531, 35.3658) -> (1.5115, 37.111)
  spline S165 degree 2 poles (-1.7759, 42.6856) (-0.8281, 43.2512) (0.9314, 42.9311) (1.3849, 42.1712) knots 0 0 0 1 2 2 2
  spline S166 degree 2 poles (1.3849, 42.1712) (1.5917, 41.8246) (1.7313, 41.2398) (1.7397, 40.9221) knots 0 0 0 1 2 2 2
  line L127 (1.7397, 40.9221) -> (1.9467, 40.9833)
  line L128 (1.9467, 40.9833) -> (2.3454, 40.3153)
  line L129 (2.3454, 40.3153) -> (-3.0364, 37.1032)
  line L130 (-3.0364, 37.1032) -> (-3.4625, 37.8172)
  line L131 (-3.4625, 37.8172) -> (-1.5419, 38.9635)
  spline S167 degree 2 poles (-1.5419, 38.9635) (-1.9252, 39.1028) (-2.5937, 39.5588) (-2.8305, 39.9554) knots 0 0 0 1 2 2 2
  spline S168 degree 2 poles (-2.8305, 39.9554) (-3.2615, 40.6777) (-2.707, 42.1299) (-1.7759, 42.6856) knots 0 0 0 1 2 2 2
  spline S169 degree 2 poles (-1.2847, 41.9765) (-1.9778, 41.5628) (-2.4194, 40.6708) (-2.1129, 40.1572) knots 0 0 0 1 2 2 2
  spline S170 degree 2 poles (-2.1129, 40.1572) (-1.9384, 39.865) (-1.3316, 39.4174) (-0.995, 39.2899) knots 0 0 0 1 2 2 2
  line L132 (-0.995, 39.2899) -> (1.222, 40.6131)
  spline S171 degree 2 poles (1.222, 40.6131) (1.1811, 40.9567) (1.0321, 41.434) (0.8826, 41.6845) knots 0 0 0 1 2 2 2
  spline S172 degree 2 poles (0.8826, 41.6845) (0.5562, 42.2315) (-0.5207, 42.4325) (-1.2847, 41.9765) knots 0 0 0 1 2 2 2
  spline S173 degree 2 poles (-4.2425, 46.9607) (-3.2655, 47.5438) (-1.5829, 47.1438) (-1.0696, 46.2837) knots 0 0 0 1 2 2 2
  spline S174 degree 2 poles (-1.0696, 46.2837) (-0.5413, 45.3986) (-1.0338, 43.7287) (-1.9774, 43.1655) knots 0 0 0 1 2 2 2
  spline S175 degree 2 poles (-1.9774, 43.1655) (-2.9461, 42.5874) (-4.642, 42.9908) (-5.1529, 43.8467) knots 0 0 0 1 2 2 2
  spline S176 degree 2 poles (-5.1529, 43.8467) (-5.6662, 44.7068) (-5.2153, 46.3801) (-4.2425, 46.9607) knots 0 0 0 1 2 2 2
  spline S177 degree 2 poles (-3.8015, 46.2217) (-4.553, 45.7732) (-4.9248, 44.7359) (-4.5934, 44.1806) knots 0 0 0 1 2 2 2
  spline S178 degree 2 poles (-4.5934, 44.1806) (-4.262, 43.6253) (-3.17, 43.456) (-2.4185, 43.9045) knots 0 0 0 1 2 2 2
  spline S179 degree 2 poles (-2.4185, 43.9045) (-1.6878, 44.3406) (-1.2976, 45.3945) (-1.629, 45.9498) knots 0 0 0 1 2 2 2
  spline S180 degree 2 poles (-1.629, 45.9498) (-1.958, 46.5009) (-3.0583, 46.6653) (-3.8015, 46.2217) knots 0 0 0 1 2 2 2
  line L133 (-4.724, 52.1602) -> (-4.2979, 51.4462)
  line L134 (-4.2979, 51.4462) -> (-4.7238, 51.1921)
  spline S181 degree 2 poles (-4.7238, 51.1921) (-4.2639, 51.0192) (-3.6362, 50.5841) (-3.4194, 50.2209) knots 0 0 0 1 2 2 2
  spline S182 degree 2 poles (-3.4194, 50.2209) (-3.2524, 49.9412) (-3.1279, 49.353) (-3.1978, 49.0621) knots 0 0 0 1 2 2 2
  spline S183 degree 2 poles (-3.1978, 49.0621) (-3.2677, 48.7713) (-3.695, 48.2444) (-4.0875, 48.0102) knots 0 0 0 1 2 2 2
  line L135 (-4.0875, 48.0102) -> (-6.5967, 46.5126)
  line L136 (-6.5967, 46.5126) -> (-7.0229, 47.2265)
  line L137 (-7.0229, 47.2265) -> (-4.8184, 48.5422)
  spline S184 degree 2 poles (-4.8184, 48.5422) (-4.5094, 48.7266) (-4.1343, 49.0185) (-4.0363, 49.1958) knots 0 0 0 1 2 2 2
  spline S185 degree 2 poles (-4.0363, 49.1958) (-3.9384, 49.3732) (-3.98, 49.7561) (-4.147, 50.0358) knots 0 0 0 1 2 2 2
  spline S186 degree 2 poles (-4.147, 50.0358) (-4.3039, 50.2988) (-4.9317, 50.7339) (-5.2749, 50.8631) knots 0 0 0 1 2 2 2
  line L138 (-5.2749, 50.8631) -> (-8.1641, 49.1388)
  line L139 (-8.1641, 49.1388) -> (-8.5902, 49.8527)
  line L140 (-8.5902, 49.8527) -> (-4.724, 52.1602)
  line L141 (-5.7756, 53.9221) -> (-5.3495, 53.2082)
  line L142 (-5.3495, 53.2082) -> (-10.7313, 49.9961)
  line L143 (-10.7313, 49.9961) -> (-11.1574, 50.7101)
  line L144 (-11.1574, 50.7101) -> (-5.7756, 53.9221)
  line L145 (-13.3447, 57.8189) -> (-8.8356, 59.0492)
  line L146 (-8.8356, 59.0492) -> (-8.4394, 58.3854)
  line L147 (-8.4394, 58.3854) -> (-10.8025, 55.5707)
  line L148 (-10.8025, 55.5707) -> (-7.2034, 56.3145)
  line L149 (-7.2034, 56.3145) -> (-6.8122, 55.659)
  line L150 (-6.8122, 55.659) -> (-10.028, 52.2618)
  line L151 (-10.028, 52.2618) -> (-10.4741, 53.0091)
  line L152 (-10.4741, 53.0091) -> (-7.9265, 55.5432)
  line L153 (-7.9265, 55.5432) -> (-11.5232, 54.7669)
  line L154 (-11.5232, 54.7669) -> (-11.8745, 55.3556)
  line L155 (-11.8745, 55.3556) -> (-9.4989, 58.1777)
  line L156 (-9.4989, 58.1777) -> (-12.9161, 57.1008)
  line L157 (-12.9161, 57.1008) -> (-13.3447, 57.8189)
  spline S187 degree 2 poles (-11.6768, 62.88) (-11.566, 62.8272) (-11.1829, 62.6595) (-11.038, 62.5591) knots 0 0 0 1 2 2 2
  spline S188 degree 2 poles (-11.038, 62.5591) (-10.834, 62.426) (-10.5262, 62.1285) (-10.3368, 61.8111) knots 0 0 0 1 2 2 2
  spline S189 degree 2 poles (-10.3368, 61.8111) (-10.1798, 61.5481) (-10.0778, 60.9692) (-10.1334, 60.6925) knots 0 0 0 1 2 2 2
  spline S190 degree 2 poles (-10.1334, 60.6925) (-10.1899, 60.4266) (-10.5354, 59.9429) (-10.7943, 59.7884) knots 0 0 0 1 2 2 2
  spline S191 degree 2 poles (-10.7943, 59.7884) (-11.1951, 59.5492) (-11.9847, 59.5819) (-12.3893, 59.8897) knots 0 0 0 1 2 2 2
  spline S192 degree 2 poles (-12.3893, 59.8897) (-12.7514, 60.1549) (-13.4447, 61.0604) (-13.8103, 61.6066) knots 0 0 0 1 2 2 2
  line L158 (-13.8103, 61.6066) -> (-13.9356, 61.5319)
  spline S193 degree 2 poles (-13.9356, 61.5319) (-14.161, 61.3973) (-14.3511, 61.08) (-14.3482, 60.8949) knots 0 0 0 1 2 2 2
  spline S194 degree 2 poles (-14.3482, 60.8949) (-14.3453, 60.7098) (-14.1586, 60.2832) (-14.034, 60.0745) knots 0 0 0 1 2 2 2
  spline S195 degree 2 poles (-14.034, 60.0745) (-13.887, 59.8282) (-13.3547, 59.2399) (-13.0259, 58.9831) knots 0 0 0 1 2 2 2
  line L159 (-13.0259, 58.9831) -> (-13.001, 58.9414)
  line L160 (-13.001, 58.9414) -> (-13.6649, 58.5451)
  spline S196 degree 2 poles (-13.6649, 58.5451) (-13.8321, 58.7115) (-14.3984, 59.3757) (-14.6152, 59.739) knots 0 0 0 1 2 2 2
  spline S197 degree 2 poles (-14.6152, 59.739) (-14.8744, 60.1732) (-15.1079, 60.8492) (-15.0896, 61.1885) knots 0 0 0 1 2 2 2
  spline S198 degree 2 poles (-15.0896, 61.1885) (-15.068, 61.5128) (-14.6999, 62.044) (-14.3366, 62.2608) knots 0 0 0 1 2 2 2
  line L161 (-14.3366, 62.2608) -> (-11.6938, 63.8381)
  line L162 (-11.6938, 63.8381) -> (-11.2677, 63.1242)
  line L163 (-11.2677, 63.1242) -> (-11.6768, 62.88)
  line L164 (-12.2196, 62.556) -> (-13.2926, 61.9156)
  spline S199 degree 2 poles (-13.2926, 61.9156) (-13.1197, 61.6734) (-12.5853, 60.9392) (-12.3739, 60.7369) knots 0 0 0 1 2 2 2
  spline S200 degree 2 poles (-12.3739, 60.7369) (-12.1252, 60.5003) (-11.5736, 60.3256) (-11.2813, 60.5) knots 0 0 0 1 2 2 2
  spline S201 degree 2 poles (-11.2813, 60.5) (-10.9473, 60.6994) (-10.8533, 61.3104) (-11.09, 61.707) knots 0 0 0 1 2 2 2
  spline S202 degree 2 poles (-11.09, 61.707) (-11.2919, 62.0452) (-11.8813, 62.4352) (-12.2196, 62.556) knots 0 0 0 1 2 2 2
  line L165 (-18.3855, 64.244) -> (-18.363, 64.2064)
  spline S203 degree 2 poles (-18.363, 64.2064) (-18.3391, 64.0904) (-18.1833, 63.6965) (-18.101, 63.5587) knots 0 0 0 1 2 2 2
  spline S204 degree 2 poles (-18.101, 63.5587) (-17.8294, 63.1036) (-17.2328, 62.9388) (-16.7484, 63.2278) knots 0 0 0 1 2 2 2
  line L166 (-16.7484, 63.2278) -> (-16.619, 63.3051)
  line L167 (-16.619, 63.3051) -> (-17.3267, 64.4908)
  line L168 (-17.3267, 64.4908) -> (-16.7881, 64.8123)
  line L169 (-16.7881, 64.8123) -> (-16.0929, 63.6474)
  line L170 (-16.0929, 63.6474) -> (-12.7653, 65.6334)
  line L171 (-12.7653, 65.6334) -> (-12.3392, 64.9195)
  line L172 (-12.3392, 64.9195) -> (-15.6668, 62.9335)
  line L173 (-15.6668, 62.9335) -> (-15.3777, 62.4492)
  line L174 (-15.3777, 62.4492) -> (-15.9163, 62.1277)
  line L175 (-15.9163, 62.1277) -> (-16.2054, 62.612)
  line L176 (-16.2054, 62.612) -> (-16.3348, 62.5348)
  spline S205 degree 2 poles (-16.3348, 62.5348) (-17.0279, 62.1211) (-18.1954, 62.4265) (-18.6066, 63.1154) knots 0 0 0 1 2 2 2
  spline S206 degree 2 poles (-18.6066, 63.1154) (-18.7237, 63.3117) (-18.9154, 63.7182) (-18.9825, 63.8877) knots 0 0 0 1 2 2 2
  line L177 (-18.9825, 63.8877) -> (-18.3855, 64.244)
  line L178 (-19.8656, 66.724) -> (-19.8432, 66.6865)
  spline S207 degree 2 poles (-19.8432, 66.6865) (-19.8193, 66.5705) (-19.6634, 66.1765) (-19.5812, 66.0388) knots 0 0 0 1 2 2 2
  spline S208 degree 2 poles (-19.5812, 66.0388) (-19.3096, 65.5837) (-18.7129, 65.4188) (-18.2286, 65.7079) knots 0 0 0 1 2 2 2
  line L179 (-18.2286, 65.7079) -> (-18.0992, 65.7851)
  line L180 (-18.0992, 65.7851) -> (-18.8069, 66.9709)
  line L181 (-18.8069, 66.9709) -> (-18.2683, 67.2923)
  line L182 (-18.2683, 67.2923) -> (-17.573, 66.1275)
  line L183 (-17.573, 66.1275) -> (-14.2454, 68.1135)
  line L184 (-14.2454, 68.1135) -> (-13.8193, 67.3995)
  line L185 (-13.8193, 67.3995) -> (-17.1469, 65.4135)
  line L186 (-17.1469, 65.4135) -> (-16.8579, 64.9292)
  line L187 (-16.8579, 64.9292) -> (-17.3965, 64.6077)
  line L188 (-17.3965, 64.6077) -> (-17.6855, 65.0921)
  line L189 (-17.6855, 65.0921) -> (-17.815, 65.0148)
  spline S209 degree 2 poles (-17.815, 65.0148) (-18.508, 64.6012) (-19.6756, 64.9066) (-20.0867, 65.5955) knots 0 0 0 1 2 2 2
  spline S210 degree 2 poles (-20.0867, 65.5955) (-20.2038, 65.7917) (-20.3955, 66.1983) (-20.4627, 66.3677) knots 0 0 0 1 2 2 2
  line L190 (-20.4627, 66.3677) -> (-19.8656, 66.724)
  spline S211 degree 2 poles (-17.0767, 71.9275) (-16.9659, 71.8747) (-16.5827, 71.7071) (-16.4379, 71.6067) knots 0 0 0 1 2 2 2
  spline S212 degree 2 poles (-16.4379, 71.6067) (-16.2339, 71.4736) (-15.926, 71.176) (-15.7367, 70.8587) knots 0 0 0 1 2 2 2
  spline S213 degree 2 poles (-15.7367, 70.8587) (-15.5797, 70.5957) (-15.4776, 70.0167) (-15.5333, 69.74) knots 0 0 0 1 2 2 2
  spline S214 degree 2 poles (-15.5333, 69.74) (-15.5898, 69.4742) (-15.9353, 68.9905) (-16.1942, 68.836) knots 0 0 0 1 2 2 2
  spline S215 degree 2 poles (-16.1942, 68.836) (-16.595, 68.5968) (-17.3846, 68.6295) (-17.7891, 68.9373) knots 0 0 0 1 2 2 2
  spline S216 degree 2 poles (-17.7891, 68.9373) (-18.1512, 69.2025) (-18.8446, 70.108) (-19.2102, 70.6542) knots 0 0 0 1 2 2 2
  line L191 (-19.2102, 70.6542) -> (-19.3354, 70.5794)
  spline S217 degree 2 poles (-19.3354, 70.5794) (-19.5609, 70.4449) (-19.7509, 70.1276) (-19.748, 69.9425) knots 0 0 0 1 2 2 2
  spline S218 degree 2 poles (-19.748, 69.9425) (-19.7451, 69.7574) (-19.5585, 69.3308) (-19.4339, 69.1221) knots 0 0 0 1 2 2 2
  spline S219 degree 2 poles (-19.4339, 69.1221) (-19.2869, 68.8757) (-18.7546, 68.2874) (-18.4258, 68.0307) knots 0 0 0 1 2 2 2
  line L192 (-18.4258, 68.0307) -> (-18.4009, 67.9889)
  line L193 (-18.4009, 67.9889) -> (-19.0647, 67.5927)
  spline S220 degree 2 poles (-19.0647, 67.5927) (-19.232, 67.7591) (-19.7983, 68.4233) (-20.0151, 68.7865) knots 0 0 0 1 2 2 2
  spline S221 degree 2 poles (-20.0151, 68.7865) (-20.2742, 69.2208) (-20.5078, 69.8967) (-20.4895, 70.2361) knots 0 0 0 1 2 2 2
  spline S222 degree 2 poles (-20.4895, 70.2361) (-20.4679, 70.5604) (-20.0997, 71.0916) (-19.7365, 71.3083) knots 0 0 0 1 2 2 2
  line L194 (-19.7365, 71.3083) -> (-17.0936, 72.8857)
  line L195 (-17.0936, 72.8857) -> (-16.6675, 72.1717)
  line L196 (-16.6675, 72.1717) -> (-17.0767, 71.9275)
  line L197 (-17.6195, 71.6036) -> (-18.6925, 70.9632)
  spline S223 degree 2 poles (-18.6925, 70.9632) (-18.5196, 70.721) (-17.9851, 69.9867) (-17.7738, 69.7845) knots 0 0 0 1 2 2 2
  spline S224 degree 2 poles (-17.7738, 69.7845) (-17.525, 69.5479) (-16.9734, 69.3732) (-16.6811, 69.5476) knots 0 0 0 1 2 2 2
  spline S225 degree 2 poles (-16.6811, 69.5476) (-16.3471, 69.7469) (-16.2532, 70.3579) (-16.4899, 70.7546) knots 0 0 0 1 2 2 2
  spline S226 degree 2 poles (-16.4899, 70.7546) (-16.6917, 71.0928) (-17.2812, 71.4827) (-17.6195, 71.6036) knots 0 0 0 1 2 2 2
  point P0 (0, 0)
  constraints: 2 other
extrude "Extrusion2" cut sketch "Sketch2" against normal blind 5
equation "\"d5\" = 0.8 * d2"
body "Solid1"
